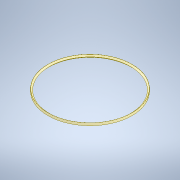
# Autodesk Inventor part: self-aligning-ring-2
Saved by Autodesk Inventor 2021 (Build 250183000, 183)
## iProperties
Created: 2020-06-29
Part Number: self-aligning-ring-2
Material: Nylon 6/6
Document SubType Name: Modeling
Density: 1.13 g/cm^3
Appearance: Nylon 6
Mass: 19.7025 g
Surface Area: 104.615 cm^2
Volume: 17.4358 cm^3
Author: MK
Subject: 100/120*5
Autodesk Inventor part; units mm, degrees
ref_plane "YZ Plane" through (0, 0, 0) normal (1, 0, 0) x (0, 1, 0)
ref_plane "XZ Plane" through (0, 0, 0) normal (0, 1, 0) x (-1, 0, 0)
ref_plane "XY Plane" through (0, 0, 0) normal (0, 0, 1) x (1, 0, 0)
sketch "Sketch1" plane through (0, 0, 0) normal (0, 0, 1) x (1, 0, 0)
  line L0 (0, 2.5713) -> (0, -2.5713)
  line L1 (-367.5, 10.75) -> (-367.5, -10.75)
  line L2 (-367.5, -10.75) -> (-364.8771, -10.75)
  line L3 (-364.8771, -10.75) -> (-355, 0)
  line L4 (-355, 0) -> (-366.7, 10.75)
  line L5 (-366.7, 10.75) -> (-367.5, 10.75)
  point P0 (0, 0)
  point P1 (0, 0)
  point P2 (-367.5, 0)
  dimension "dimensionA_parameter" = 0.8
  dimension "dimensionD_parameter" = 21.5
  dimension "d0" = 90
  dimension "fasciaCollaudo2_parameter" = 12.5
  dimension "externalDiameter2_parameter" = 735
  dimension "d1" = 710
  constraints: 12 end point, 2 coincident, 2 horizontal alignment, 2 midpoint, 2 vertical, 1 parallel, 1 perpendicular
  measures "dimensionA_parameter" distance of L4.end L1.start
  measures "dimensionD_parameter" distance of L1.start L1.end
  measures "d0" angle of L3 L4
  measures "fasciaCollaudo2_parameter" distance from line of L1 L3.end
  measures "externalDiameter2_parameter" diameter of L1 L0
  measures "d1" diameter of L3.end L0
revolve "Revolution4" add sketch "Sketch1" angle 360 about axis through (0, 2.5713, 0) along (0, -1, 0)
body "Solid4"
